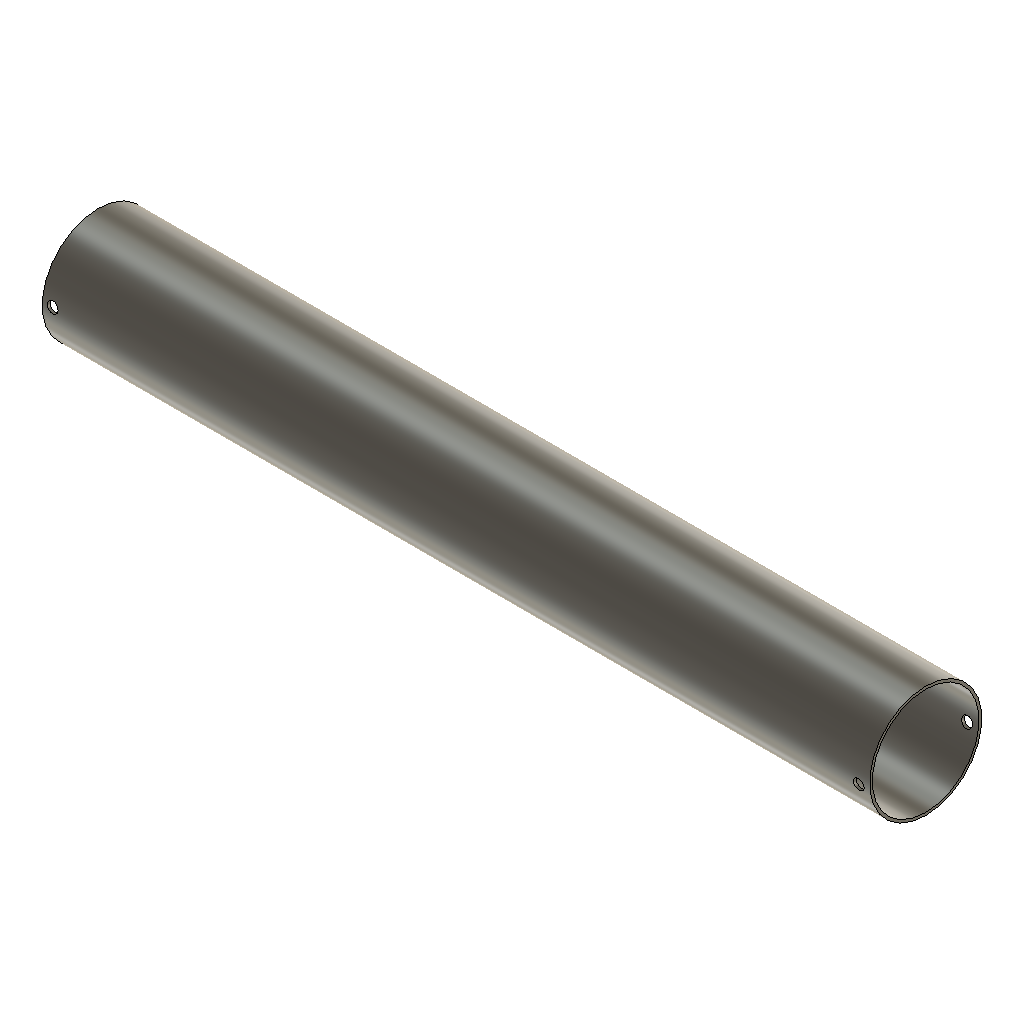
handle (Autodesk Fusion 360 design; units mm, degrees)
part number: 2026-09-04-00-00-18-277
Autodesk Fusion 360 part; units mm, degrees
note: some values were not read from the file. Set by a fixed rule: which face or edge a step refers to.
sketch "Sketch2" plane through (0, 0, 0) normal (0, 0, 1) x (1, 0, 0)
  circle A0 centre (0, 0) radius 10.5
  dimension "d15" = 21
  constraint coincident A0.centre origin
  measures "d15" diameter of A0
extrude "Extrude3" add sketch "Sketch2" along normal blind 100
extrude "Extrude4" add 1 faces at (-2.9623, 1.0316, 100) along direction (0, 0, 1) blind 55
shell "Shell4" thickness 0.5 removed faces 1 at (-2.9623, 1.0316, 155)
sketch "Sketch3" plane through (0, 0, 0) normal (0, 1, 0) x (1, 0, 0)
  line L0 (1.8551, -103.1591) -> (-4.1449, -103.1591)
  line L1 (-4.1449, -103.1591) -> (-4.1449, -77.5591)
  line L2 (-4.1449, -77.5591) -> (1.8551, -77.5591)
  line L3 (1.8551, -77.5591) -> (1.8551, -103.1591)
  dimension "d21" = 6
  dimension "d22" = 25.6
  constraint horizontal L0
  constraint vertical L1
  constraint horizontal L2
  constraint vertical L3
  measures "d21" distance of L0.start L0.end
  measures "d22" distance of L0.start L2.end
extrude "Extrude5" cut sketch "Sketch3" along normal blind 19
move_body "Move1" bodies 1 to x (0, 0, -1) y (0, 1, 0) z (1, 0, 0) at (-77.5, 0, 77.5)
extrude "Extrude6" cut 1 faces at (-77, 3.5886, 75.2736) along direction (-1, 0, 0) blind 1
sketch "Sketch4" plane through (0, 0, 0) normal (0, 1, 0) x (1, 0, 0)
  circle A0 centre (75.3676, -76.1708) radius 1
  dimension "d27" = 2
  measures "d27" diameter of A0
extrude "Extrude7" cut sketch "Sketch4" along normal blind 21
mirror "Mirror1" about plane through (0, 0, 0) normal (0, 1, 0) of "Extrude7"
sketch "Sketch5" plane through (0, 0, 0) normal (0, 1, 0) x (1, 0, 0)
  circle A0 centre (-75.5671, -78.134) radius 1
  dimension "d32" = 2
  measures "d32" diameter of A0
extrude "Extrude8" cut sketch "Sketch5" along normal blind 19
mirror "Mirror2" about plane through (0, 0, 0) normal (0, 1, 0) of "Extrude8"
